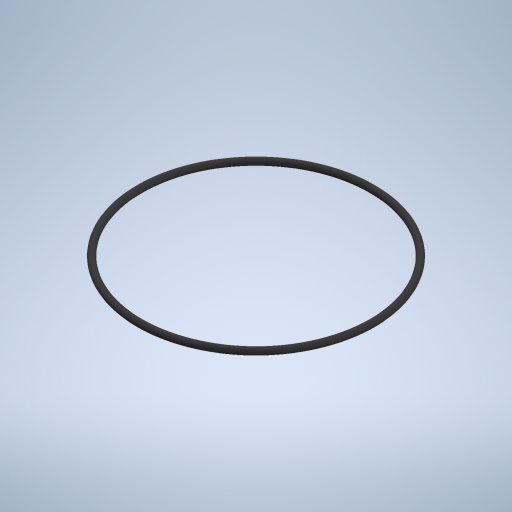
# Autodesk Inventor part: 2.62
Saved by Autodesk Inventor 2024.3 (Build 283343000, 343)
## iProperties
Created: 2024-12-23
Part Number: 2.62
Material: Caucho
Document SubType Name: Modeling
Designer: Usuario
Density: 0.93 g/cm^3
Appearance: Caucho - Negro
Author: Usuario
Autodesk Inventor part; units mm, degrees
ref_plane "YZ Plane" through (0, 0, 0) normal (1, 0, 0) x (0, 1, 0)
ref_plane "XZ Plane" through (0, 0, 0) normal (0, 1, 0) x (-1, 0, 0)
ref_plane "XY Plane" through (0, 0, 0) normal (0, 0, 1) x (1, 0, 0)
sketch "Boceto1" plane through (0, 0, 0) normal (0, 0, 1) x (1, 0, 0)
  circle A0 centre (45.595, 0) radius 1.31
  line L0 (0, -22.1425) -> (0, 22.1425)
  line L1 (0, 0) -> (45.595, 0) construction
  point P0 (44.285, 0)
  dimension "d0" = 2.62
  dimension "d3" = 44.285
  constraints: 4 end point, 1 horizontal, 1 horizontal alignment, 1 midpoint, 1 perpendicular, 1 point on line, 2 other
  measures "d3" distance of L1.start point (44.285, 0)
revolve "Revolución1" add sketch "Boceto1" angle 360 about axis through (0, -22.1425, 0) along (0, 1, 0)
